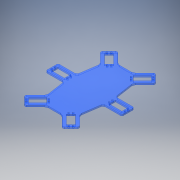
# Autodesk Inventor part: Upper Chassis Plate
Saved by Autodesk Inventor 2016 (Build 200138000, 138)
## iProperties
Created: 2016-05-22
Part Number: Upper Chassis Plate
Material: Polycarbonate, Smoke
Document SubType Name: Modeling
Designer: Jacob
Density: 1.2 g/cm^3
Appearance: Clear - Blue
Author: Jacob
Autodesk Inventor part; units mm, degrees
ref_plane "YZ Plane" through (0, 0, 0) normal (1, 0, 0) x (0, 1, 0)
ref_plane "XZ Plane" through (0, 0, 0) normal (0, 1, 0) x (-1, 0, 0)
ref_plane "XY Plane" through (0, 0, 0) normal (0, 0, 1) x (1, 0, 0)
sketch "Sketch1" plane through (0, 0, 0) normal (0, 1, 0) x (-1, 0, 0)
  line L0 (45, 105) -> (-45, 105)
  line L1 (-45, 105) -> (-45, -105)
  line L2 (-45, -105) -> (45, -105)
  line L3 (45, -105) -> (45, 105)
  line L4 (45, 105) -> (-45, -105) construction
  line L5 (-45, 105) -> (45, -105) construction
  line L6 (-45, 0) -> (-70, 0)
  line L7 (45, 0) -> (70, 0)
  line L8 (45, -105) -> (30.504, -105)
  line L9 (45, -105) -> (45, -90.504)
  line L10 (45, 105) -> (45, 90.504)
  line L11 (45, 105) -> (30.504, 105)
  line L12 (-45, 105) -> (-30.504, 105)
  line L13 (-45, 105) -> (-45, 90.504)
  line L14 (-45, -105) -> (-45, -90.504)
  line L15 (-45, -105) -> (-30.504, -105)
  line L16 (-30.504, -105) -> (-45, -90.504)
  line L17 (-45, 90.504) -> (-30.504, 105)
  line L18 (45, 90.504) -> (30.504, 105)
  line L19 (45, -90.504) -> (30.504, -105)
  line L20 (-30.504, -105) -> (-59.1418, -133.6378)
  line L21 (-30.504, -105) -> (9.996, -105) construction
  line L22 (-59.1418, -133.6378) -> (-73.6375, -119.1421)
  line L23 (-73.6375, -119.1421) -> (-45, -90.504)
  line L24 (-70, 0) -> (-70, -10.25)
  line L25 (-70, -10.25) -> (-110.5, -10.25)
  line L26 (-110.5, -10.25) -> (-110.5, 10.25)
  line L27 (-110.5, 10.25) -> (-70, 10.25)
  line L28 (-70, 10.25) -> (-70, 0)
  line L29 (-45, 90.504) -> (-73.6378, 119.1418)
  line L30 (-45, 90.504) -> (-4.5, 90.504) construction
  line L31 (-73.6378, 119.1418) -> (-59.1421, 133.6375)
  line L32 (-59.1421, 133.6375) -> (-30.5046, 105)
  line L33 (45, 90.504) -> (73.6378, 119.1418)
  line L34 (45, 90.504) -> (85.5, 90.504) construction
  line L35 (73.6378, 119.1418) -> (59.1421, 133.6375)
  line L36 (59.1421, 133.6375) -> (30.5046, 105)
  line L37 (45, -90.504) -> (73.6378, -119.1418)
  line L38 (45, -90.504) -> (85.5, -90.504) construction
  line L39 (73.6378, -119.1418) -> (59.1421, -133.6375)
  line L40 (59.1421, -133.6375) -> (30.504, -105)
  line L41 (70, 0) -> (70, -10.25)
  line L42 (70, -10.25) -> (110.5, -10.25)
  line L43 (110.5, -10.25) -> (110.5, 10.25)
  line L44 (110.5, 10.25) -> (70, 10.25)
  line L45 (70, 10.25) -> (70, 0)
  line L46 (119.5, -19.25) -> (61, -19.25)
  line L47 (61, -19.25) -> (61, 0)
  line L48 (61, 0) -> (61, 19.25)
  line L49 (61, 19.25) -> (119.5, 19.25)
  line L50 (119.5, 19.25) -> (119.5, -19.25)
  line L51 (51.364, -84.14) -> (86.3657, -119.1418)
  line L52 (86.3657, -119.1418) -> (59.1422, -146.3654)
  line L53 (59.1422, -146.3654) -> (24.1401, -111.364)
  line L54 (-24.14, -111.364) -> (-59.1418, -146.3657)
  line L55 (-59.1418, -146.3657) -> (-86.3654, -119.1422)
  line L56 (-86.3654, -119.1422) -> (-51.364, -84.1401)
  line L57 (-119.5, -19.25) -> (-61, -19.25)
  line L58 (-61, -19.25) -> (-61, 0)
  line L59 (-61, 0) -> (-61, 19.25)
  line L60 (-61, 19.25) -> (-119.5, 19.25)
  line L61 (-119.5, 19.25) -> (-119.5, -19.25)
  line L62 (-51.364, 84.14) -> (-86.3657, 119.1418)
  line L63 (-86.3657, 119.1418) -> (-59.1421, 146.3654)
  line L64 (-59.1421, 146.3654) -> (-24.1407, 111.364)
  line L65 (24.1407, 111.364) -> (59.1421, 146.3654)
  line L66 (59.1421, 146.3654) -> (86.3657, 119.1418)
  line L67 (86.3657, 119.1418) -> (51.364, 84.1401)
  line L68 (51.364, -84.14) -> (61, -19.25)
  line L69 (24.1401, -111.364) -> (-24.1401, -111.364)
  line L70 (-51.364, -84.1401) -> (-61, -19.25)
  line L71 (-61, 19.25) -> (-51.364, 84.14)
  line L72 (24.1407, 111.364) -> (-24.1407, 111.364)
  line L73 (51.364, 84.1401) -> (61, 19.25)
  point P0 (0, 0)
  dimension "d0" = 90
  dimension "d1" = 210
  dimension "d2" = 25
  dimension "d3" = 25
  dimension "d4" = 14.496
  dimension "d5" = 14.496
  dimension "d6" = 14.496
  dimension "d7" = 14.496
  dimension "d8" = 14.496
  dimension "d9" = 14.496
  dimension "d10" = 14.496
  dimension "d11" = 14.496
  dimension "d12" = 40.5
  dimension "d13" = 135
  dimension "d14" = 20.5
  dimension "d15" = 10.25
  dimension "d16" = 40.5
  dimension "d17" = 20.5
  dimension "d18" = 40.5
  dimension "d19" = 40.5
  dimension "d20" = 135
  dimension "d21" = 20.5
  dimension "d22" = 40.5
  dimension "d23" = 45
  dimension "d24" = 20.5
  dimension "d25" = 40.5
  dimension "d26" = 45
  dimension "d27" = 20.5
  dimension "d28" = 10.25
  dimension "d29" = 40.5
  dimension "d30" = 20.5
  dimension "d31" = 9
  dimension "d32" = 9
  dimension "d33" = 9
  dimension "d34" = 9
  dimension "d35" = 9
  dimension "d36" = 9
  constraints: 148 end point, 25 perpendicular, 12 point on line, 10 horizontal, 6 parallel, 4 equal length, 4 midpoint, 2 vertical, 16 other
  measures "d0" distance of L2.end L1.end
  measures "d1" distance of L1.end L0.end
  measures "d2" distance of L6.start L6.end
  measures "d3" distance of L7.start L7.end
  measures "d4" distance of L2.end L8.end
  measures "d5" distance of L2.end L9.end
  measures "d6" distance of L0.start L10.end
  measures "d7" distance of L0.start L11.end
  measures "d8" distance of L0.end L12.end
  measures "d9" distance of L0.end L13.end
  measures "d10" distance of L1.end L14.end
  measures "d11" distance of L1.end L15.end
  measures "d12" distance of L15.end L20.end
  measures "d13" angle of L20 L21
  measures "d14" distance of L20.end L22.end
  measures "d15" distance of L6.end L24.end
  measures "d16" distance of L24.end L25.end
  measures "d17" distance of L25.end L26.end
  measures "d18" distance of L26.end L27.end
  measures "d19" distance of L13.end L29.end
  measures "d20" angle of L30 L29
  measures "d21" distance of L29.end L31.end
  measures "d22" distance of L10.end L33.end
  measures "d23" angle of L34 L33
  measures "d24" distance of L33.end L35.end
  measures "d25" distance of L9.end L37.end
  measures "d26" angle of L37 L38
  measures "d27" distance of L37.end L39.end
  measures "d28" distance of L7.end L41.end
  measures "d29" distance of L41.end L42.end
  measures "d30" distance of L42.end L43.end
  measures "d31" distance between parallel lines of L42 L46
  measures "d32" distance between parallel lines of L37 L51
  measures "d33" distance between parallel lines of L20 L54
  measures "d34" distance between parallel lines of L25 L57
  measures "d35" distance between parallel lines of L29 L62
  measures "d36" distance between parallel lines of L36 L65
extrude "Extrusion1" add sketch "Sketch1" along normal blind 5 contours L18 L3 L19 L2 L16 L1 L17 L0 | L0 L32 L31 L29 L1 L6 L59 L71 L62 L63 L64 L72 L65 L66 L67 L73 L48 L7 L3 L33 L35 L36 | L7 L47 L68 L51 L52 L53 L69 L54 L55 L56 L70 L58 L6 L1 L23 L22 L20 L2 L40 L39 L37 L3 | L48 L49 L50 L46 L47 | L58 L57 L61 L60 L59
sketch "Sketch2" plane through (0, 5, 0) normal (0, 1, 0) x (1, 0, 0)
  line L0 (-30.504, -105) -> (-30.5046, -105) projected
  line L1 (-30.5046, -105) -> (-59.1421, -133.6375) projected
  line L2 (-59.1421, -133.6375) -> (-73.6378, -119.1418) projected
  line L3 (-73.6378, -119.1418) -> (-45, -90.504) projected
  line L4 (-45, -90.504) -> (-30.504, -105) projected
  line L5 (-45, 90.504) -> (-73.6378, 119.1418) projected
  line L6 (-73.6378, 119.1418) -> (-59.1421, 133.6375) projected
  line L7 (-59.1421, 133.6375) -> (-30.504, 105) projected
  line L8 (-30.504, 105) -> (-45, 90.504) projected
  line L9 (30.504, 105) -> (59.1418, 133.6378) projected
  line L10 (59.1418, 133.6378) -> (73.6375, 119.1421) projected
  line L11 (73.6375, 119.1421) -> (45, 90.504) projected
  line L12 (45, 90.504) -> (30.504, 105) projected
  line L13 (70, 10.25) -> (110.5, 10.25) projected
  line L14 (110.5, 10.25) -> (110.5, -10.25) projected
  line L15 (110.5, -10.25) -> (70, -10.25) projected
  line L16 (70, -10.25) -> (70, 10.25) projected
  line L17 (-70, -10.25) -> (-110.5, -10.25) projected
  line L18 (-110.5, -10.25) -> (-110.5, 10.25) projected
  line L19 (-110.5, 10.25) -> (-70, 10.25) projected
  line L20 (-70, 10.25) -> (-70, -10.25) projected
  line L21 (-119.5, 19.25) -> (-119.5, -19.25) projected
  line L22 (-119.5, -19.25) -> (-61, -19.25) projected
  line L23 (-61, -19.25) -> (-51.364, -84.1401) projected
  line L24 (-51.364, -84.1401) -> (-86.3657, -119.1418) projected
  line L25 (-86.3657, -119.1418) -> (-59.1421, -146.3654) projected
  line L26 (-59.1421, -146.3654) -> (-24.1407, -111.364) projected
  line L27 (-24.1407, -111.364) -> (24.1407, -111.364) projected
  line L28 (24.1407, -111.364) -> (59.1421, -146.3654) projected
  line L29 (59.1421, -146.3654) -> (86.3657, -119.1418) projected
  line L30 (86.3657, -119.1418) -> (51.364, -84.14) projected
  line L31 (51.364, -84.14) -> (61, -19.25) projected
  line L32 (61, -19.25) -> (119.5, -19.25) projected
  line L33 (119.5, -19.25) -> (119.5, 19.25) projected
  line L34 (119.5, 19.25) -> (61, 19.25) projected
  line L35 (61, 19.25) -> (51.364, 84.1401) projected
  line L36 (51.364, 84.1401) -> (86.3654, 119.1422) projected
  line L37 (86.3654, 119.1422) -> (59.1418, 146.3657) projected
  line L38 (59.1418, 146.3657) -> (24.1401, 111.364) projected
  line L39 (24.1401, 111.364) -> (-24.1401, 111.364) projected
  line L40 (-24.1401, 111.364) -> (-59.1422, 146.3654) projected
  line L41 (-59.1422, 146.3654) -> (-86.3657, 119.1418) projected
  line L42 (-86.3657, 119.1418) -> (-51.364, 84.14) projected
  line L43 (-51.364, 84.14) -> (-61, 19.25) projected
  line L44 (-61, 19.25) -> (-119.5, 19.25) projected
  line L45 (30.504, -105) -> (45, -90.504) projected
  line L46 (45, -90.504) -> (73.6378, -119.1418) projected
  line L47 (73.6378, -119.1418) -> (59.1421, -133.6375) projected
  line L48 (59.1421, -133.6375) -> (30.5046, -105) projected
  line L49 (30.5046, -105) -> (30.504, -105) projected
  line L50 (-226.8598, -181.3552) -> (-267.3598, -181.3552)
  line L51 (-267.3598, -181.3552) -> (-267.3598, -160.8552)
  line L52 (-267.3598, -160.8552) -> (-226.8598, -160.8552)
  line L53 (-226.8598, -160.8552) -> (-226.8598, -181.3552)
  line L54 (-267.3598, -171.1052) -> (-271.8598, -171.1052)
  line L55 (-226.8598, -171.1052) -> (-222.3598, -171.1052)
  line L56 (-222.3598, -171.1052) -> (-222.3598, -166.1052)
  line L57 (-222.3598, -171.1052) -> (-222.3598, -176.1052)
  line L58 (-271.8598, -171.1052) -> (-271.8598, -166.1052)
  line L59 (-271.8598, -171.1052) -> (-271.8598, -176.1052)
  circle A0 centre (-271.8598, -166.1052) radius 2.5
  circle A1 centre (-271.8598, -176.1052) radius 2.5
  circle A2 centre (-222.3598, -166.1052) radius 2.5
  circle A3 centre (-222.3598, -176.1052) radius 2.5
  line L60 (-226.8598, -62.722) -> (-255.4976, -34.0841)
  line L61 (-255.4976, -34.0841) -> (-241.002, -19.5884)
  line L62 (-241.002, -19.5884) -> (-212.3641, -48.2263)
  line L63 (-212.3641, -48.2263) -> (-226.8598, -62.722)
  line L64 (-248.2498, -26.8363) -> (-251.4318, -23.6543)
  line L65 (-251.4318, -23.6543) -> (-247.8962, -20.1188)
  line L66 (-251.4318, -23.6543) -> (-254.9673, -27.1898)
  circle A4 centre (-247.8962, -20.1188) radius 2.5
  circle A5 centre (-254.9673, -27.1898) radius 2.5
  line L67 (-224.2263, 83.9693) -> (-252.8641, 55.3315)
  line L68 (-252.8641, 55.3315) -> (-267.3598, 69.8272)
  line L69 (-267.3598, 69.8272) -> (-238.722, 98.465)
  line L70 (-238.722, 98.465) -> (-224.2263, 83.9693)
  line L71 (-260.112, 62.5793) -> (-263.294, 59.3973)
  line L72 (-263.294, 59.3973) -> (-266.8295, 62.9329)
  line L73 (-263.294, 59.3973) -> (-259.7584, 55.8618)
  circle A6 centre (-266.8295, 62.9329) radius 2.5
  circle A7 centre (-259.7584, 55.8618) radius 2.5
  line L74 (-219.612, -55.4741) -> (-216.43, -58.6561)
  line L75 (-219.612, -55.4741) -> (-215.112, -55.4741) construction
  line L76 (-216.43, -58.6561) -> (-219.9655, -62.1916)
  line L77 (-216.43, -58.6561) -> (-211.43, -58.6561) construction
  line L78 (-216.43, -58.6561) -> (-212.8945, -55.1206)
  line L79 (-216.43, -58.6561) -> (-211.43, -58.6561) construction
  circle A8 centre (-219.612, -61.8381) radius 2.5
  circle A9 centre (-212.8945, -55.1206) radius 2.5
  line L80 (-231.4742, 91.2171) -> (-228.2922, 94.3991)
  line L81 (-231.4742, 91.2171) -> (-226.9742, 91.2171) construction
  line L82 (-228.2922, 94.3991) -> (-231.8277, 97.9347)
  line L83 (-228.2922, 94.3991) -> (-224.7566, 90.8636)
  circle A10 centre (-224.7566, 90.8636) radius 2.5
  circle A11 centre (-231.8277, 97.9347) radius 2.5
  line L84 (-110.5, 10.25) -> (-110.5, -10.25) projected
  line L85 (-73.6378, 119.1418) -> (-45, 90.504) projected
  line L86 (-59.1421, -133.6375) -> (-30.5046, -105) projected
  line L87 (73.6378, -119.1418) -> (45, -90.504) projected
  line L88 (70, 10.25) -> (70, -10.25) projected
  line L89 (110.5, 10.25) -> (70, 10.25) projected
  line L90 (45, 90.504) -> (73.6375, 119.1421) projected
  line L91 (45, 90.504) -> (30.504, 105) projected
  line L92 (59.1418, 133.6378) -> (30.504, 105) projected
  line L93 (-70, -10.25) -> (-110.5, -10.25)
  line L94 (-110.5, -10.25) -> (-110.5, 10.25)
  line L95 (-110.5, 10.25) -> (-70, 10.25)
  line L96 (-70, 10.25) -> (-70, -10.25)
  line L97 (-110.5, 0) -> (-115, 0)
  line L98 (-70, 0) -> (-65.5, 0)
  line L99 (-65.5, 0) -> (-65.5, 5)
  line L100 (-65.5, 0) -> (-65.5, -5)
  line L101 (-115, 0) -> (-115, 5)
  line L102 (-115, 0) -> (-115, -5)
  circle A12 centre (-115, 5) radius 2.5
  circle A13 centre (-115, -5) radius 2.5
  circle A14 centre (-65.5, 5) radius 2.5
  circle A15 centre (-65.5, -5) radius 2.5
  line L103 (110.5, -10.25) -> (70, -10.25)
  line L104 (70, -10.25) -> (70, 10.25)
  line L105 (70, 10.25) -> (110.5, 10.25)
  line L106 (110.5, 10.25) -> (110.5, -10.25)
  line L107 (70, 0) -> (65.5, 0)
  line L108 (110.5, 0) -> (115, 0)
  line L109 (115, 0) -> (115, 5)
  line L110 (115, 0) -> (115, -5)
  line L111 (65.5, 0) -> (65.5, 5)
  line L112 (65.5, 0) -> (65.5, -5)
  circle A16 centre (65.5, 5) radius 2.5
  circle A17 centre (65.5, -5) radius 2.5
  circle A18 centre (115, 5) radius 2.5
  circle A19 centre (115, -5) radius 2.5
  line L113 (-73.6378, 119.1418) -> (-59.1421, 133.6375)
  line L114 (-66.39, 126.3897) -> (-69.572, 129.5716)
  line L115 (-69.572, 129.5716) -> (-66.0364, 133.1072)
  line L116 (-69.572, 129.5716) -> (-73.1075, 126.0361)
  circle A20 centre (-66.0364, 133.1072) radius 2.5
  circle A21 centre (-73.1075, 126.0361) radius 2.5
  line L117 (-59.1421, 133.6375) -> (-30.5043, 104.9997)
  line L118 (-45, 90.504) -> (-73.6378, 119.1418)
  line L119 (-30.5043, 104.9997) -> (-45, 90.504)
  line L120 (-37.7522, 97.7518) -> (-34.5702, 94.5699)
  line L121 (-37.7522, 97.7518) -> (-33.2522, 97.7518) construction
  line L122 (-34.5702, 94.5699) -> (-38.1057, 91.0343)
  line L123 (-34.5702, 94.5699) -> (-29.5702, 94.5699) construction
  line L124 (-34.5702, 94.5699) -> (-31.0346, 98.1054)
  line L125 (-34.5702, 94.5699) -> (-29.5702, 94.5699) construction
  circle A22 centre (-37.7522, 91.3879) radius 2.5
  circle A23 centre (-31.0346, 98.1054) radius 2.5
  line L126 (30.5043, -104.9997) -> (45, -90.504)
  line L127 (37.7522, -97.7518) -> (34.5702, -94.5699)
  line L128 (34.5702, -94.5699) -> (38.1057, -91.0343)
  line L129 (34.5702, -94.5699) -> (31.0346, -98.1054)
  circle A24 centre (38.1057, -91.0343) radius 2.5
  circle A25 centre (31.0346, -98.1054) radius 2.5
  line L130 (45, -90.504) -> (73.6378, -119.1418)
  line L131 (59.1421, -133.6375) -> (30.5043, -104.9997)
  line L132 (73.6378, -119.1418) -> (59.1421, -133.6375)
  line L133 (66.39, -126.3897) -> (69.572, -129.5716)
  line L134 (66.39, -126.3897) -> (70.89, -126.3897) construction
  line L135 (69.572, -129.5716) -> (66.0364, -133.1072)
  line L136 (69.572, -129.5716) -> (74.572, -129.5716) construction
  line L137 (69.572, -129.5716) -> (73.1075, -126.0361)
  line L138 (69.572, -129.5716) -> (74.572, -129.5716) construction
  circle A26 centre (66.39, -132.7536) radius 2.5
  circle A27 centre (73.1075, -126.0361) radius 2.5
  line L139 (-59.1421, -133.6375) -> (-73.6378, -119.1418)
  line L140 (-66.39, -126.3897) -> (-69.572, -129.5716)
  line L141 (-69.572, -129.5716) -> (-73.1075, -126.0361)
  line L142 (-69.572, -129.5716) -> (-66.0364, -133.1072)
  circle A28 centre (-73.1075, -126.0361) radius 2.5
  circle A29 centre (-66.0364, -133.1072) radius 2.5
  line L143 (-73.6378, -119.1418) -> (-45, -90.504)
  line L144 (-30.5043, -104.9997) -> (-59.1421, -133.6375)
  line L145 (-45, -90.504) -> (-30.5043, -104.9997)
  line L146 (-37.7522, -97.7518) -> (-34.5702, -94.5699)
  line L147 (-37.7522, -97.7518) -> (-33.2522, -97.7518) construction
  line L148 (-34.5702, -94.5699) -> (-38.1057, -91.0343)
  line L149 (-34.5702, -94.5699) -> (-31.0346, -98.1054)
  circle A30 centre (-31.0346, -98.1054) radius 2.5
  circle A31 centre (-38.1057, -91.0343) radius 2.5
  line L150 (45, 90.504) -> (30.5043, 104.9997)
  line L151 (37.7522, 97.7518) -> (34.5702, 94.5699)
  line L152 (34.5702, 94.5699) -> (31.0346, 98.1054)
  line L153 (34.5702, 94.5699) -> (38.1057, 91.0343)
  circle A32 centre (31.0346, 98.1054) radius 2.5
  circle A33 centre (38.1057, 91.0343) radius 2.5
  line L154 (30.5043, 104.9997) -> (59.1421, 133.6375)
  line L155 (73.6378, 119.1418) -> (45, 90.504)
  line L156 (59.1421, 133.6375) -> (73.6378, 119.1418)
  line L157 (66.39, 126.3897) -> (69.572, 129.5716)
  line L158 (66.39, 126.3897) -> (70.89, 126.3897) construction
  line L159 (69.572, 129.5716) -> (66.0364, 133.1072)
  line L160 (69.572, 129.5716) -> (73.1075, 126.0361)
  circle A34 centre (73.1075, 126.0361) radius 2.5
  circle A35 centre (66.0364, 133.1072) radius 2.5
  point P0 (0, 0)
  dimension "d39" = 40.5
  dimension "d40" = 20.5
  dimension "d41" = 4.5
  dimension "d42" = 4.5
  dimension "d43" = 5
  dimension "d44" = 5
  dimension "d45" = 5
  dimension "d46" = 5
  dimension "d47" = 5
  dimension "d48" = 5
  dimension "d49" = 5
  dimension "d50" = 5
  dimension "d51" = 40.5
  dimension "d52" = 20.5
  dimension "d53" = 4.5
  dimension "d57" = 5
  dimension "d58" = 5
  dimension "d59" = 5
  dimension "d60" = 5
  dimension "d63" = 40.5
  dimension "d64" = 20.5
  dimension "d65" = 4.5
  dimension "d69" = 5
  dimension "d70" = 5
  dimension "d71" = 5
  dimension "d72" = 5
  dimension "d75" = 4.5
  dimension "d76" = 45
  dimension "d78" = 5
  dimension "d79" = 135
  dimension "d80" = 5
  dimension "d81" = 45
  dimension "d82" = 5
  dimension "d83" = 5
  dimension "d84" = 4.5
  dimension "d85" = 45
  dimension "d86" = 5
  dimension "d87" = 90
  dimension "d88" = 5
  dimension "d89" = 5
  dimension "d90" = 5
  dimension "d91" = 40.5
  dimension "d92" = 20.5
  dimension "d93" = 4.5
  dimension "d94" = 4.5
  dimension "d95" = 5
  dimension "d96" = 5
  dimension "d97" = 5
  dimension "d98" = 5
  dimension "d99" = 5
  dimension "d100" = 5
  dimension "d101" = 5
  dimension "d102" = 5
  dimension "d103" = 40.5
  dimension "d104" = 20.5
  dimension "d105" = 4.5
  dimension "d106" = 4.5
  dimension "d107" = 5
  dimension "d108" = 5
  dimension "d109" = 5
  dimension "d110" = 5
  dimension "d111" = 5
  dimension "d112" = 5
  dimension "d113" = 5
  constraints: 204 end point, 57 coincident, 36 centre point, 21 horizontal, 21 parallel, 18 midpoint, 15 perpendicular, 12 equal length, 9 vertical, 3 point on line
  measures "d39" distance of L51.end L52.end
  measures "d40" distance of L50.end L51.end
  measures "d41" distance of L54.start L54.end
  measures "d42" distance of L55.start L55.end
  measures "d43" distance of L55.end L56.end
  measures "d44" distance of L55.end L57.end
  measures "d45" distance of L54.end L58.end
  measures "d46" distance of L54.end L59.end
  measures "d47" diameter of A0
  measures "d48" diameter of A1
  measures "d49" diameter of A2
  measures "d50" diameter of A3
  measures "d51" distance of L61.end L62.end
  measures "d52" distance of L61.start L61.end
  measures "d53" distance of L64.start L64.end
  measures "d57" distance of L64.end L65.end
  measures "d58" distance of L64.end L66.end
  measures "d59" diameter of A4
  measures "d60" diameter of A5
  measures "d63" distance of L68.end L69.end
  measures "d64" distance of L68.start L68.end
  measures "d65" distance of L71.start L71.end
  measures "d69" distance of L71.end L72.end
  measures "d70" distance of L71.end L73.end
  measures "d71" diameter of A6
  measures "d72" diameter of A7
  measures "d75" distance of L74.start L74.end
  measures "d76" angle of L74 L75
  measures "d78" distance of L74.end L76.end
  measures "d79" angle of L76 L77
  measures "d80" distance of L74.end L78.end
  measures "d81" angle of L79 L78
  measures "d82" diameter of A8
  measures "d83" diameter of A9
  measures "d84" distance of L80.start L80.end
  measures "d85" angle of L81 L80
  measures "d86" distance of L80.end L82.end
  measures "d87" angle of L82 L80
  measures "d88" distance of L80.end L83.end
  measures "d89" diameter of A10
  measures "d90" diameter of A11
  measures "d91" distance of L95.start L96.start
  measures "d92" distance of L93.end L95.start
  measures "d93" distance of L97.start L97.end
  measures "d94" distance of L98.start L100.start
  measures "d95" distance of L100.start L99.end
  measures "d96" distance of L100.start L100.end
  measures "d97" distance of L97.end L101.end
  measures "d98" distance of L97.end L102.end
  measures "d99" diameter of A12
  measures "d100" diameter of A13
  measures "d101" diameter of A14
  measures "d102" diameter of A15
  measures "d103" distance of L105.start L106.start
  measures "d104" distance of L103.end L105.start
  measures "d105" distance of L107.start L107.end
  measures "d106" distance of L108.start L110.start
  measures "d107" distance of L110.start L109.end
  measures "d108" distance of L110.start L110.end
  measures "d109" distance of L107.end L111.end
  measures "d110" distance of L107.end L112.end
  measures "d111" diameter of A16
  measures "d112" diameter of A17
  measures "d113" diameter of A18
extrude "Extrusion2" cut sketch "Sketch2" against normal blind 10 contours A29 | A28 | A31 | A30 | A21 | A20 | A23 | A22 | A35 | A34 | A33 | A32 | A18 | A19 | A17 | A16 | A13 | A12 | A14 | A15 | A25 | A24 | A27 | A26
fillet "Fillet1" radius 5 12 edges at (-59.1421, 2.5, 146.3654) (-86.3657, 2.5, 119.1418) (59.1421, 2.5, 146.3654) (86.3657, 2.5, 119.1418) (119.5, 2.5, 19.25) (119.5, 2.5, -19.25) (86.3654, 2.5, -119.1422) (59.1418, 2.5, -146.3657) (-59.1422, 2.5, -146.3654) (-86.3657, 2.5, -119.1418) (-119.5, 2.5, -19.25) (-119.5, 2.5, 19.25)
chamfer "Chamfer1" distance 5 angle 45 12 edges at (-24.1407, 2.5, 111.364) (24.1407, 2.5, 111.364) (51.364, 2.5, 84.14) (61, 2.5, 19.25) (61, 2.5, -19.25) (51.364, 2.5, -84.1401) (24.1401, 2.5, -111.364) (-24.1401, 2.5, -111.364) (-51.364, 2.5, -84.14) (-61, 2.5, -19.25) (-61, 2.5, 19.25) (-51.364, 2.5, 84.1401)
body "Solid1"
